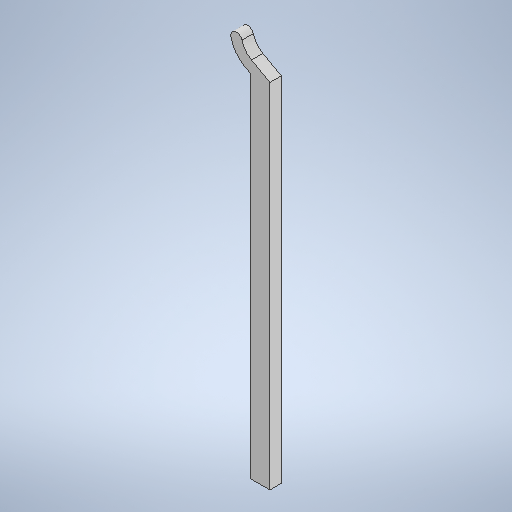
# Autodesk Inventor part: Moving Ramp Holder Shaft
Saved by Autodesk Inventor 2025.1 (Build 291241020, 241B)
## iProperties
Created: 2024-10-26
Part Number: Moving Ramp Holder Shaft
Material: Generic
Document SubType Name: Modeling
Designer: aly_g
Density: 1 g/cm^3
Appearance: Default
Author: aly_g
Autodesk Inventor part; units mm, degrees
ref_plane "YZ Plane" through (0, 0, 0) normal (1, 0, 0) x (0, 1, 0)
ref_plane "XZ Plane" through (0, 0, 0) normal (0, 1, 0) x (-1, 0, 0)
ref_plane "XY Plane" through (0, 0, 0) normal (0, 0, 1) x (1, 0, 0)
sketch "Sketch1" plane through (0, 0, 0) normal (0, 0, 1) x (1, 0, 0)
  line L0 (0, 0) -> (5, 0)
  line L1 (5, 0) -> (5, 95)
  line L2 (5, 95) -> (2.5, 95)
  line L3 (0, 92.4007) -> (0, 0)
  arc A0 (-2.5, 100) -> (2.5, 95) centre (2.5, 100) ccw
  arc A1 (-5.5, 100) -> (0, 92.4007) centre (2.5, 100) ccw
  line L4 (-5.5, 100) -> (-2.5, 100)
  point P0 (2.5, 0)
  dimension "d1" = 95
  dimension "d5" = 10
  dimension "d6" = 3
  dimension "d7" = 3
  dimension "d8" = 5
  constraints: 10 end point, 4 point on circle, 2 centre point, 2 horizontal, 2 parallel, 2 vertical alignment, 1 midpoint, 1 perpendicular
  measures "d1" distance of L0.end L1.end
  measures "d5" diameter of A0
  measures "d6" radial gap between concentric circles of A0 A1
  measures "d7" distance of L4.end L4.start
  measures "d8" distance between parallel lines of L1 L3
extrude "Extrusion1" add sketch "Sketch1" along normal blind 3
fillet "Fillet2" radius 1.5 2 edges at (-2.5, 100, 1.5) (-5.5, 100, 1.5)
sketch "Sketch3" plane through (0, 0, 3) normal (0, 0, 1) x (1, 0, 0)
  line L0 (0, 95.6699) -> (5, 92.9)
  line L1 (5, 92.9) -> (5, 95)
  line L2 (5, 95) -> (0, 95.6699)
  arc A0 (-2.365, 98.8462) -> (2.5, 95) centre (2.5, 100) ccw projected
  point P0 (0, 0)
  point P1 (0, 92.4007)
  dimension "d12" = 5
  dimension "d14" = 2.1
  constraints: 6 end point, 1 point on circle, 1 vertical, 1 vertical alignment
  measures "d12" horizontal distance of L1.end L0.start
  measures "d14" distance of L0.end L1.end
extrude "Extrusion2" cut sketch "Sketch3" against normal through all
body "Solid1"
